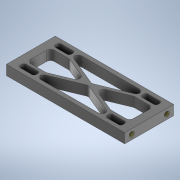
# Autodesk Inventor part: BackLink_diagonal
Saved by Autodesk Inventor 2022.3 (Build 263350000, 350)
## iProperties
Part Number: BackLink_diagonal
Material: アルミニウム 2014-T4
Document SubType Name: Modeling
Designer: Masato Kubotera
Density: 2.8 g/cm^3
Appearance: Smooth - Black
Description: A2017 T5
Mass: 8.35665 g
Surface Area: 38.6511 cm^2
Volume: 2.98452 cm^3
Author: MasatoKubotera
Autodesk Inventor part; units mm, degrees
ref_plane "YZ Plane" through (0, 0, 0) normal (1, 0, 0) x (0, 1, 0)
ref_plane "XZ Plane" through (0, 0, 0) normal (0, 1, 0) x (-1, 0, 0)
ref_plane "XY Plane" through (0, 0, 0) normal (0, 0, 1) x (1, 0, 0)
sketch "スケッチ1" plane through (0, 0, 0) normal (1, 0, 0) x (0, 1, 0)
  line L0 (-30.25, 12.5) -> (30.25, 12.5)
  line L1 (30.25, 12.5) -> (30.25, -12.5)
  line L2 (30.25, -12.5) -> (-30.25, -12.5)
  line L3 (-30.25, -12.5) -> (-30.25, 12.5)
  line L4 (-30.25, 12.5) -> (30.25, -12.5) construction
  line L5 (30.25, 12.5) -> (-30.25, -12.5) construction
  line L6 (30.25, 9) -> (26.25, 9) construction
  line L7 (26.25, 10.5) -> (26.25, 7.5) construction
  line L8 (26.25, 7.5) -> (30.25, 7.5) construction
  line L9 (26.25, 10.5) -> (30.25, 10.5) construction
  line L10 (0, 12.5) -> (0, -12.5)
  line L11 (-30.25, 0) -> (30.25, 0) construction
  line L12 (30.25, -9) -> (26.25, -9) construction
  line L13 (26.25, -10.5) -> (26.25, -7.5) construction
  line L14 (26.25, -7.5) -> (30.25, -7.5) construction
  line L15 (26.25, -10.5) -> (30.25, -10.5) construction
  line L16 (26.25, 1.5) -> (26.25, -1.5) construction
  line L17 (26.25, -1.5) -> (30.25, -1.5) construction
  line L18 (26.25, 1.5) -> (30.25, 1.5) construction
  line L19 (19.15, 10.5) -> (25.25, 10.5)
  line L20 (26.25, 9.5) -> (26.25, 8.5)
  line L21 (25.25, 7.5) -> (19.15, 7.5)
  line L22 (18.15, 8.5) -> (18.15, 9.5)
  line L23 (18.15, 10.5) -> (26.25, 7.5) construction
  line L24 (26.25, 10.5) -> (18.15, 7.5) construction
  arc A0 (19.15, 10.5) -> (18.15, 9.5) centre (19.15, 9.5) ccw
  arc A1 (18.15, 8.5) -> (19.15, 7.5) centre (19.15, 8.5) ccw
  arc A2 (25.25, 7.5) -> (26.25, 8.5) centre (25.25, 8.5) ccw
  arc A3 (26.25, 9.5) -> (25.25, 10.5) centre (25.25, 9.5) ccw
  line L25 (24.25, 6) -> (16.8808, 6)
  line L26 (16.117, 5.8484) -> (6.437, 1.8484)
  line L27 (24.25, -6) -> (16.8808, -6)
  line L28 (16.117, -5.8484) -> (6.437, -1.8484)
  line L29 (26.25, 4) -> (26.25, -4)
  line L30 (16.65, 8.5) -> (16.65, 9.0293)
  line L31 (15.4138, 7.1809) -> (0.7638, 1.1271)
  line L32 (-16.65, 8.5) -> (-16.65, 9.0293)
  line L33 (-15.4138, 7.1809) -> (-0.7638, 1.1271)
  line L34 (-14.65, 10.5) -> (14.65, 10.5)
  arc A4 (-14.65, 10.5) -> (-16.65, 8.5) centre (-14.65, 8.5) ccw
  arc A5 (-16.65, 9.0293) -> (-15.4138, 7.1809) centre (-14.65, 9.0293) ccw
  arc A6 (-0.7638, 1.1271) -> (0.7638, 1.1271) centre (0, 2.9755) ccw
  arc A7 (15.4138, 7.1809) -> (16.65, 9.0293) centre (14.65, 9.0293) ccw
  arc A8 (16.65, 8.5) -> (14.65, 10.5) centre (14.65, 8.5) ccw
  arc A9 (16.8808, 6) -> (16.117, 5.8484) centre (16.8808, 4) ccw
  arc A10 (6.437, 1.8484) -> (6.437, -1.8484) centre (7.2008, 0) ccw
  arc A11 (16.117, -5.8484) -> (16.8808, -6) centre (16.8808, -4) ccw
  arc A12 (24.25, -6) -> (26.25, -4) centre (24.25, -4) ccw
  arc A13 (26.25, 4) -> (24.25, 6) centre (24.25, 4) ccw
  line L35 (16.65, -8.5) -> (16.65, -9.0293)
  line L36 (15.4138, -7.1809) -> (0.7638, -1.1271)
  line L37 (-16.65, -8.5) -> (-16.65, -9.0293)
  line L38 (-15.4138, -7.1809) -> (-0.7638, -1.1271)
  line L39 (-14.65, -10.5) -> (14.65, -10.5)
  arc A14 (-16.65, -8.5) -> (-14.65, -10.5) centre (-14.65, -8.5) ccw
  arc A15 (-15.4138, -7.1809) -> (-16.65, -9.0293) centre (-14.65, -9.0293) ccw
  arc A16 (0.7638, -1.1271) -> (-0.7638, -1.1271) centre (0, -2.9755) ccw
  arc A17 (16.65, -9.0293) -> (15.4138, -7.1809) centre (14.65, -9.0293) ccw
  arc A18 (14.65, -10.5) -> (16.65, -8.5) centre (14.65, -8.5) ccw
  line L40 (19.15, -10.5) -> (25.25, -10.5)
  line L41 (26.25, -9.5) -> (26.25, -8.5)
  line L42 (25.25, -7.5) -> (19.15, -7.5)
  line L43 (18.15, -8.5) -> (18.15, -9.5)
  arc A19 (18.15, -9.5) -> (19.15, -10.5) centre (19.15, -9.5) ccw
  arc A20 (19.15, -7.5) -> (18.15, -8.5) centre (19.15, -8.5) ccw
  arc A21 (26.25, -8.5) -> (25.25, -7.5) centre (25.25, -8.5) ccw
  arc A22 (25.25, -10.5) -> (26.25, -9.5) centre (25.25, -9.5) ccw
  point P0 (0, 0)
  point P1 (26.25, 0)
  point P2 (22.2, 9)
  point P3 (26.25, 6)
  point P4 (16.4839, 6)
  point P5 (1.9639, 0)
  point P6 (26.25, -6)
  point P7 (16.4839, -6)
  point P8 (16.65, 10.5)
  point P9 (16.65, 7.6917)
  point P10 (0, 0.8115)
  point P11 (-16.65, 10.5)
  point P12 (-16.65, 7.6917)
  point P13 (0, -10.5)
  point P14 (0, 10.5)
  point P15 (0, 0.9755)
  point P16 (0, -0.9755)
  point P17 (16.6324, -8.7646)
  point P18 (16.6324, 8.7646)
  point P19 (-16.6324, 8.7646)
  point P20 (-16.6324, -8.7646)
  dimension "d0" = 60.5
  dimension "d1" = 25
  dimension "d2" = 4
  dimension "d3" = 3
  dimension "d5" = 3
  dimension "d6" = 18
  dimension "d8" = 1
  dimension "d10" = 2
  dimension "d11" = 1.5
  dimension "d12" = 1.5
  dimension "d13" = 1.5
  dimension "d14" = 2
  constraints: 88 end point, 46 point on circle, 37 point on line, 37 symmetric about line, 28 tangent, 23 centre point, 12 equal radius, 11 midpoint, 6 parallel, 6 perpendicular, 5 horizontal, 4 collinear, 4 vertical, 10 other
  measures "d0" distance of L0.start L0.end
  measures "d1" distance of L0.end L1.end
  measures "d2" distance of L6.end L6.start
  measures "d3" distance of L7.start L7.end
  measures "d5" distance of L18.start L17.start
  measures "d6" distance of L12.start L6.start
  measures "d8" radius of A0
  measures "d10" distance between parallel lines of L0 L19
  measures "d11" distance between parallel lines of L25 L21
  measures "d12" distance between parallel lines of L26 L31
  measures "d13" distance between parallel lines of L30 L22
  measures "d14" radius of A4
extrude "押し出し1" add sketch "スケッチ1" along normal blind 5 contours A7 L30 A8 | A18 L35 A17 | L0 L1 L2 L10 L39 A18 A17 L36 A16 A6 L31 A7 A8 L34
sketch "スケッチ2" plane through (0, 30.25, 12.5) normal (0, 1, 0) x (1, 0, 0)
  line L0 (5, 25) -> (5, 0) projected
  line L1 (5, 3.5) -> (0, 3.5) construction
  line L2 (0, 25) -> (0, 0) projected
  line L3 (5, 21.5) -> (0, 21.5) construction
  line L4 (5, 3.5) -> (0, 3.5) construction
  point P0 (2.5, 3.5)
  point P1 (2.5, 21.5)
  point P2 (2.5, 21.5)
  point P3 (2.5, 3.5)
  constraints: 6 end point, 4 point on line, 3 horizontal, 3 midpoint, 2 coincident
hole "穴1" at (2.5, 30.25, -9) at (2.5, 30.25, 9) direction (0, -1, 0) diameter 2.459 depth 5 thread size "M3x0.5" class "6H" standard "ISO Metric profile"
mirror "ミラー1" about plane through (0, 0, -10.5) normal (0, -1, 0)
equation "\"d13\" = d11"
